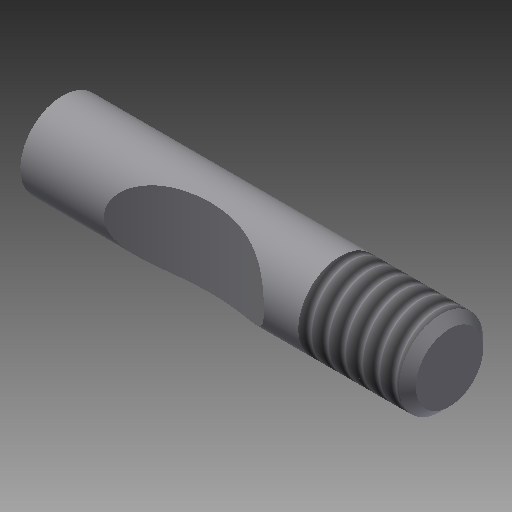
# Autodesk Inventor part: Screw Lock
Saved by Autodesk Inventor 2017 (Build 210142000, 142)
## iProperties
Created: 2012-08-06
Part Number: Screw Lock
Material: Generic
Document SubType Name: Modeling
Designer: John
Density: 1 g/cm^3
Appearance: Default
Author: John
Autodesk Inventor part; units mm, degrees
ref_plane "YZ Plane" through (0, 0, 0) normal (1, 0, 0) x (0, 1, 0)
ref_plane "XZ Plane" through (0, 0, 0) normal (0, 1, 0) x (-1, 0, 0)
ref_plane "XY Plane" through (0, 0, 0) normal (0, 0, 1) x (1, 0, 0)
sketch "Sketch1" plane through (0, 0, 0) normal (1, 0, 0) x (0, 1, 0)
  circle A0 centre (0, 0) radius 1.9685
  dimension "d0" = 3.937
  constraints: 1 centre point, 1 coincident
  measures "d0" diameter of A0
extrude "Extrusion1" add sketch "Sketch1" along normal blind 18.034
thread "Thread1" size "8-32 UNC" class "2A" standard "ANSI Unified Screw Threads" length 5.08
sketch "Sketch2" plane through (0, 0, 0) normal (0, 1, 0) x (-1, 0, 0)
  line L0 (-18.034, 1.9685) -> (0, 1.9685) projected
  line L1 (0, 1.9685) -> (0, -1.9685) projected
  line L2 (0, -1.9685) -> (-18.034, -1.9685) projected
  line L3 (-18.034, -1.9685) -> (-18.034, 1.9685) projected
  circle A0 centre (-7.62, 6.9469) radius 6.223
  point P0 (0, 0)
  dimension "d6" = 7.62
  dimension "d7" = 4.9784
  dimension "d8" = 12.446
  constraints: 1 centre point
  measures "d6" distance from line of L1 A0.centre
  measures "d7" distance from line of L0 A0.centre
  measures "d8" diameter of A0
extrude "Extrusion2" cut sketch "Sketch2" along normal through all both and the other way through all contours A0 L0 | L0 A0
chamfer "Chamfer1" distance 0.3969 angle 45 1 edges at (18.034, -1.9685, 0)
body "Solid1"
